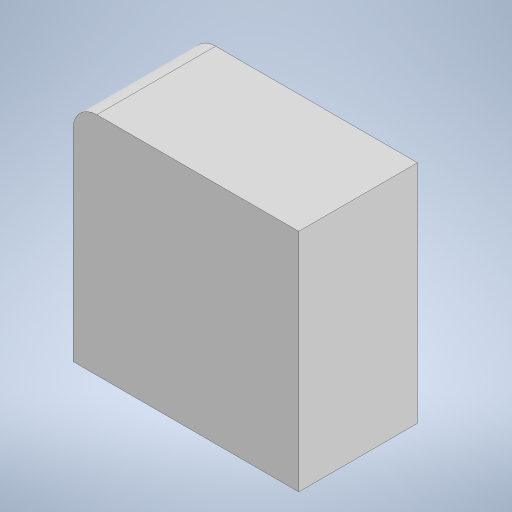
# Autodesk Inventor part: pied_coque
Saved by Autodesk Inventor 2023 (Build 270158000, 158)
## iProperties
Created: 2023-03-28
Part Number: pied_coque
Material: Générique
Document SubType Name: Modeling
Designer: egozi
Density: 1 g/cm^3
Appearance: Par défaut
Author: egozi
Autodesk Inventor part; units mm, degrees
ref_plane "YZ Plane" through (0, 0, 0) normal (1, 0, 0) x (0, 1, 0)
ref_plane "XZ Plane" through (0, 0, 0) normal (0, 1, 0) x (-1, 0, 0)
ref_plane "XY Plane" through (0, 0, 0) normal (0, 0, 1) x (1, 0, 0)
sketch "Esquisse1" plane through (0, 0, 0) normal (0, 0, 1) x (1, 0, 0)
  line L0 (0, -1.8) -> (0, 10.8) projected
  line L1 (-10.8, 0) -> (1.8, 0) projected
  line L2 (0, 0) -> (-9, 0)
  line L3 (-9, 0) -> (-9, 9)
  line L4 (-9, 9) -> (0, 9)
  line L5 (0, 9) -> (0, 0)
  point P0 (0, 9)
  dimension "d0" = 9
  dimension "d1" = 9
  constraints: 8 end point, 2 parallel, 1 horizontal, 1 perpendicular
  measures "d0" distance of L3.end L4.end
  measures "d1" distance of L2.end L3.end
extrude "Extrusion1" add sketch "Esquisse1" along normal blind 1.8
sketch "Esquisse2" plane through (0, 0, 1.8) normal (0, 0, 1) x (1, 0, 0)
  line L0 (-14, 14) -> (5, 14)
  line L1 (5, 14) -> (5, -5)
  line L2 (5, -5) -> (-14, -5)
  line L3 (-14, -5) -> (-14, 14)
  line L4 (-9, 9) -> (-9, 0) projected
  line L5 (0, 9) -> (-9, 9) projected
  line L6 (0, 0) -> (0, 9) projected
  line L7 (-9, 0) -> (0, 0) projected
  dimension "d4" = 5
  dimension "d5" = 5
  dimension "d6" = 5
  dimension "d7" = 5
  constraints: 8 end point, 2 parallel, 1 horizontal, 1 perpendicular
  measures "d4" distance between parallel lines of L3 L4
  measures "d5" distance between parallel lines of L5 L0
  measures "d6" distance between parallel lines of L6 L1
  measures "d7" distance between parallel lines of L7 L2
extrude "Extrusion2" add sketch "Esquisse2" along normal blind 10 contours L0 L1 L2 L3 | L5 L6 L7 L4
fillet "Congé1" radius 2 1 edges at (-14, 14, 6.8)
